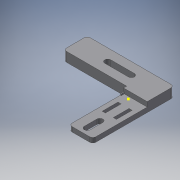
# Autodesk Inventor part: FiberMount
Saved by Autodesk Inventor 2019 (Build 230136000, 136)
## iProperties
Created: 2019-05-24
Part Number: FiberMount
Material: Generic
Document SubType Name: Modeling
Designer: aorfi
Density: 1 g/cm^3
Appearance: Default
Author: aorfi
Autodesk Inventor part; units mm, degrees
ref_plane "YZ Plane" through (0, 0, 0) normal (1, 0, 0) x (0, 1, 0)
ref_plane "XZ Plane" through (0, 0, 0) normal (0, 1, 0) x (-1, 0, 0)
ref_plane "XY Plane" through (0, 0, 0) normal (0, 0, 1) x (1, 0, 0)
sketch "Sketch1" plane through (0, 0, 0) normal (0, 1, 0) x (-1, 0, 0)
  line L0 (-7.5, 30) -> (7.5, 30)
  line L1 (7.5, 30) -> (7.5, -21.5)
  line L2 (7.5, -21.5) -> (-7.5, -21.5)
  line L3 (-7.5, -21.5) -> (-7.5, 30)
  line L4 (7.5, -21.5) -> (47.5, -21.5)
  line L5 (47.5, -6.5) -> (7.5, -6.5)
  line L6 (47.5, -6.5) -> (47.5, -21.5)
  point P0 (0, 0)
  point P1 (0, -21.5)
  dimension "d30" = 15
  dimension "d31" = 21.5
  dimension "d32" = 30
  dimension "d61" = 15
  dimension "d91" = 40
  constraints: 14 end point, 3 horizontal, 2 parallel, 1 midpoint, 1 perpendicular, 1 point on line, 1 vertical, 1 vertical alignment
  measures "d30" distance of L0.start L0.end
  measures "d31" distance from line of L2 point (0, 0)
  measures "d32" distance from line of point (0, 0) L0
  measures "d61" distance between parallel lines of L4 L5
  measures "d91" distance between parallel lines of L1 L6
extrude "Extrusion1" add sketch "Sketch1" along normal mid plane 3
sketch "Sketch4" plane through (0, 1.5, 0) normal (0, 1, 0) x (1, 0, 0)
  line L0 (7.5, 4.5) -> (-7.5, 4.5)
  line L1 (7.5, 4.5) -> (7.5, 14.5)
  line L2 (-7.5, 6.5) -> (-7.5, 4.5)
  line L3 (7.5, -30) -> (7.5, 21.5) projected
  line L4 (-7.5, 6.5) -> (-7.5, -30) projected
  line L5 (-7.5, -30) -> (7.5, -30) projected
  line L6 (7.5, 21.5) -> (-47.5, 21.5) projected
  line L7 (7.5, 21.5) -> (-7.5, 21.5)
  line L8 (-7.5, -30) -> (7.5, -30) projected
  line L9 (7.5, -30) -> (7.5, 21.5) projected
  line L10 (7.5, 21.5) -> (-47.5, 21.5) projected
  line L11 (-47.5, 6.5) -> (-7.5, 6.5) projected
  line L12 (-7.5, 6.5) -> (-7.5, -30) projected
  line L13 (-47.5, 21.5) -> (-47.5, 6.5) projected
  point P0 (0, 0)
  dimension "d89" = 2
  constraints: 8 end point, 2 collinear, 2 horizontal, 2 other
  measures "d89" distance between parallel lines of L11 L0
extrude "Extrusion3" add sketch "Sketch4" along normal blind 3 contours L0 L2 L11 L13 L6 L3 L1
sketch "Sketch5" plane through (0, 1.5, 0) normal (0, 1, 0) x (1, 0, 0)
  line L0 (-2.5, -12) -> (-4.5, -12)
  line L1 (-4.5, -12) -> (-4.5, -2)
  line L2 (-4.5, -2) -> (-2.5, -2)
  line L3 (-2.5, -2) -> (-2.5, -12)
  line L4 (-2.5, -12) -> (-4.5, -2) construction
  line L5 (-4.5, -12) -> (-2.5, -2) construction
  line L6 (4.5, -12) -> (2.5, -12)
  line L7 (2.5, -12) -> (2.5, -2)
  line L8 (2.5, -2) -> (4.5, -2)
  line L9 (4.5, -2) -> (4.5, -12)
  line L10 (4.5, -12) -> (2.5, -2) construction
  line L11 (2.5, -12) -> (4.5, -2) construction
  line L12 (-3.5, -7) -> (3.5, -7) construction
  line L13 (-7.5, 4.5) -> (7.5, 4.5) projected
  point P0 (0, 0)
  point P1 (0, -7)
  dimension "d24" = 2
  dimension "d25" = 10
  dimension "d26" = 7
  dimension "d90" = 6.5
  constraints: 26 end point, 5 midpoint, 4 parallel, 3 horizontal, 2 equal length, 2 perpendicular, 1 point on line, 1 vertical alignment
  measures "d24" distance of L7.end L8.end
  measures "d25" distance of L8.end L6.start
  measures "d26" distance of L12.start L12.end
  measures "d90" distance between parallel lines of L2 L13
extrude "Extrusion4" cut sketch "Sketch5" against normal blind 2
sketch "Sketch6" plane through (0, 1.5, 0) normal (0, 1, 0) x (1, 0, 0)
  circle A0 centre (0, -18) radius 1.8986
  circle A1 centre (0, -26) radius 1.8986
  line L0 (1.8986, -26) -> (1.8986, -18)
  line L1 (-1.8986, -26) -> (-1.8986, -18)
  line L2 (-7.5, -30) -> (7.5, -30) projected
  point P0 (0, 0)
  dimension "d33" = 3.7973
  dimension "d36" = 3.7973
  dimension "d37" = 8
  dimension "d68" = 4
  constraints: 4 end point, 4 point on circle, 3 tangent, 2 centre point, 2 vertical alignment, 1 vertical
  measures "d33" diameter of A0
  measures "d36" diameter of A1
  measures "d37" distance of A0.centre A1.centre
  measures "d68" distance from line of A1.centre L2
extrude "Extrusion5" cut sketch "Sketch6" against normal through all
fillet "Fillet2" radius 2 3 edges at (7.5, 1.5, -21.5) (7.5, 0, 30) (-7.5, 0, 30)
sketch "Sketch8" plane through (0, 1.5, 0) normal (0, 1, 0) x (1, 0, 0)
  line L0 (-7.5, 4.5) -> (7.5, 4.5) projected
  line L1 (-7.5, 4.5) -> (-7, 4.5)
  line L2 (-7, 4.5) -> (-7, 2.5)
  line L3 (-7, 2.5) -> (-7.5, 2.5)
  line L4 (-7.5, 2.5) -> (-7.5, 4.5)
  point P0 (0, 0)
  dimension "d74" = 0.5
  dimension "d75" = 2
  constraints: 8 end point, 2 parallel, 1 horizontal, 1 perpendicular
  measures "d74" distance of L2.end L3.end
  measures "d75" distance of L1.end L2.end
extrude "Extrusion6" add sketch "Sketch8" along normal blind 1
sketch "Sketch10" plane through (0, 4.5, 0) normal (0, 1, 0) x (1, 0, 0)
  point P0 (0, 0)
sketch "Sketch11" plane through (0, 4.5, 0) normal (0, 1, 0) x (1, 0, 0)
  circle A0 centre (-27, 14) radius 1.8986
  circle A1 centre (-12, 14) radius 1.8987
  line L0 (-27, 12.1014) -> (-12, 12.1014)
  line L1 (-27, 15.8986) -> (-12, 15.8986)
  line L2 (-19.5, 6.5) -> (-19.5, 21.5) construction
  line L3 (5.5, 21.5) -> (-47.5, 21.5) construction
  line L4 (-47.5, 6.5) -> (-7.5, 6.5) projected
  line L5 (-7.5, 6.5) -> (-7.5, 4.5) projected
  point P0 (0, 0)
  point P1 (-19.5, 14)
  point P2 (-42.5, 21.5)
  point P3 (-19.5, 15.8986)
  dimension "d85" = 3.7973
  dimension "d86" = 15
  dimension "d92" = 12
  constraints: 6 end point, 4 point on circle, 4 tangent, 3 point on line, 2 centre point, 2 horizontal, 2 midpoint, 1 horizontal alignment, 1 vertical
  measures "d85" diameter of A0
  measures "d86" distance of A1.centre A0.centre
  measures "d92" distance between parallel lines of L5 L2
extrude "Extrusion7" cut sketch "Sketch11" against normal blind 10
sketch "Sketch12" plane through (0, -1.5, 0) normal (0, 1, 0) x (1, 0, 0)
  circle A0 centre (-39.5, 14) radius 6.477
  line L0 (-47.5, 6.5) -> (-7.5, 6.5) construction
  line L1 (-39.5, 6.5) -> (-39.5, 21.5) construction
  line L2 (5.5, 21.5) -> (-47.5, 21.5) construction
  line L3 (-47.5, 6.5) -> (-47.5, 21.5) construction
  point P0 (0, 0)
  point P1 (-42.5, 21.5)
  point P2 (-47.5, 16.5)
  dimension "d93" = 12.954
  dimension "d96" = 8
  constraints: 2 end point, 2 point on line, 1 centre point, 1 coincident, 1 midpoint, 1 vertical
  measures "d93" diameter of A0
  measures "d96" distance between parallel lines of L3 L1
extrude "Extrusion8" cut sketch "Sketch12" along normal blind 4.7625
fillet "Fillet3" radius 2 1 edges at (-47.5, 1.5, -6.5)
equation "\"d36\" = d33"
body "Solid1"
